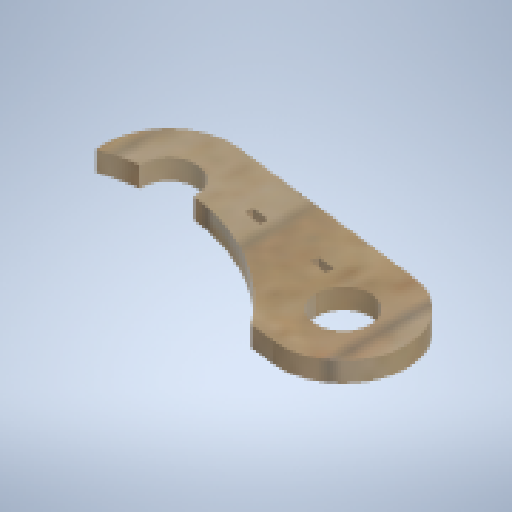
# Autodesk Inventor part: gear_plate_2
Saved by Autodesk Inventor 2024.1 (Build 281209000, 209)
## iProperties
Created: 2024-04-01
Part Number: gear_plate_2
Material: 木材 (カエデ材)
Document SubType Name: Modeling
Designer: hibik
Density: 0.67 g/cm^3
Appearance: ナチュラル カエデ材 - 光沢 濃い着色
Author: hibik
Autodesk Inventor part; units mm, degrees
ref_plane "YZ Plane" through (0, 0, 0) normal (1, 0, 0) x (0, 1, 0)
ref_plane "XZ Plane" through (0, 0, 0) normal (0, 1, 0) x (-1, 0, 0)
ref_plane "XY Plane" through (0, 0, 0) normal (0, 0, 1) x (1, 0, 0)
sketch "スケッチ1" plane through (0, 0, 0) normal (0, 1, 0) x (-1, 0, 0)
  line L0 (25, 0) -> (-25, 0)
  line L1 (-25, 0) -> (-25, -107)
  line L2 (-25, -107) -> (25, -107)
  line L3 (25, -107) -> (25, 0)
  circle A0 centre (0, 0) radius 25
  circle A1 centre (0, 0) radius 57 construction
  circle A2 centre (0, -82) radius 25
  circle A3 centre (0, 0) radius 75 construction
  circle A4 centre (0, -82) radius 10.75
  circle A5 centre (0, 0) radius 10
  circle A6 centre (0, 0) radius 82
  circle A7 centre (-78.9027, -72.2729) radius 25
  circle A8 centre (-78.9027, -72.2729) radius 10.75
  line L4 (-78.9027, -72.2729) -> (-81.9615, -97.085)
  line L5 (-81.9615, -97.085) -> (-3.0588, -106.8122)
  line L6 (3.0588, -57.1878) -> (-75.8438, -47.4607)
  point P0 (25, -78.0961)
  point P1 (10.7269, -81.2954)
  point P2 (-10.7269, -81.2954)
  point P3 (-25, -78.0961)
  point P4 (-65.9901, -48.6755)
  point P5 (25, -82)
  dimension "d0" = 114
  dimension "d2" = 150
  dimension "d3" = 21.5
  dimension "d4" = 20
  dimension "d5" = 50
  dimension "d13" = 79.5
  constraints: 14 end point, 8 centre point, 8 coincident, 8 tangent, 5 point on circle, 2 equal radius, 2 parallel, 2 perpendicular, 1 horizontal, 1 midpoint, 1 vertical alignment, 4 other
  measures "d0" diameter of A1
  measures "d2" diameter of A3
  measures "d3" diameter of A4
  measures "d4" diameter of A5
  measures "d5" distance of L1.end L2.end
  measures "d13" distance from line of A2.centre L4
extrude "押し出し1" add sketch "スケッチ1" along normal blind 8 contours L3 A2 A6 | A2 A6 A4 | A6 A7 L6 | A6 A2 L1 | L1 L5 A7 A6 | L5 L1 A2 | A7 picked at (-16.5005, -84.9893)
sketch "スケッチ3" plane through (0, 8, 0) normal (0, 1, 0) x (1, 0, 0)
  line L0 (62.1118, 99.5321) -> (61.1193, 99.6545)
  line L1 (61.1193, 99.6545) -> (60.997, 98.662)
  line L2 (60.997, 98.662) -> (61.9894, 98.5396)
  line L3 (61.9894, 98.5396) -> (62.1118, 99.5321)
  line L4 (32.3372, 103.2027) -> (31.3447, 103.3251)
  line L5 (31.3447, 103.3251) -> (31.2224, 102.3326)
  line L6 (31.2224, 102.3326) -> (32.2148, 102.2102)
  line L7 (32.2148, 102.2102) -> (32.3372, 103.2027)
  line L8 (81.9615, 97.085) -> (3.0588, 106.8122) projected
  point P0 (0, 0)
  dimension "d14" = 30
  dimension "d15" = 20
  dimension "d16" = 1
  dimension "d17" = 1
  constraints: 16 end point, 5 collinear, 4 parallel, 2 perpendicular
  measures "d14" distance between parallel lines of L5 L1
  measures "d15" distance from line of L8.start L3
  measures "d16" distance from line of L1 L2.end
  measures "d17" distance between parallel lines of L8 L2
extrude "押し出し3" cut sketch "スケッチ3" against normal through all
sketch "スケッチ4" plane through (0, 8, 0) normal (0, 1, 0) x (1, 0, 0)
  line L0 (81.9615, 97.085) -> (17.0947, 105.0818) projected
  line L1 (63.2539, 84.2777) -> (56.3065, 85.1342)
  line L2 (56.3065, 85.1342) -> (55.9395, 82.1568)
  line L3 (55.9395, 82.1568) -> (62.8869, 81.3003)
  line L4 (62.8869, 81.3003) -> (63.2539, 84.2777)
  line L5 (33.4794, 87.9484) -> (26.5319, 88.8048)
  line L6 (26.5319, 88.8048) -> (26.1649, 85.8274)
  line L7 (26.1649, 85.8274) -> (33.1123, 84.9709)
  line L8 (33.1123, 84.9709) -> (33.4794, 87.9484)
  line L9 (61.9894, 98.5396) -> (60.997, 98.662) projected
  line L10 (32.2148, 102.2102) -> (31.2224, 102.3326) projected
  line L11 (61.4932, 98.6008) -> (59.7802, 84.706)
  line L12 (31.7186, 102.2714) -> (30.0056, 88.3766)
  point P0 (0, 0)
  dimension "d21" = 7
  dimension "d22" = 15
  dimension "d23" = 3
  constraints: 20 end point, 6 perpendicular, 4 midpoint, 4 parallel, 3 collinear
  measures "d21" distance between parallel lines of L2 L4
  measures "d22" distance between parallel lines of L0 L1
  measures "d23" distance between parallel lines of L1 L3
extrude "押し出し4" cut sketch "スケッチ4" against normal through all
